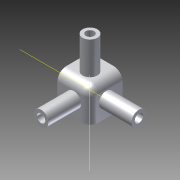
# Autodesk Inventor part: Corner
Saved by Autodesk Inventor 2011 (Build 150239000, 239)
## iProperties
Created: 2011-07-18
Part Number: Corner
Document SubType Name: Modeling
Designer: Seb Madgwick
Density: 1 g/cm^3
Author: Seb Madgwick
Autodesk Inventor part; units mm, degrees
ref_plane "YZ Plane" through (0, 0, 0) normal (1, 0, 0) x (0, 1, 0)
ref_plane "XZ Plane" through (0, 0, 0) normal (0, 1, 0) x (-1, 0, 0)
ref_plane "XY Plane" through (0, 0, 0) normal (0, 0, 1) x (1, 0, 0)
sketch "Sketch1" plane through (0, 0, 0) normal (0, 0, 1) x (1, 0, 0)
  line L0 (10, 10) -> (10, -10)
  line L1 (10, 10) -> (-10, 10)
  line L2 (-10, 10) -> (-10, -10)
  line L3 (-10, -10) -> (10, -10)
  point P0 (0, 0)
  dimension "d2" = 20
  dimension "d3" = 20
  dimension "d4" = 10
  dimension "d5" = 10
  constraints: 8 end point, 2 perpendicular, 1 parallel
  measures "d2" distance of L0.start L0.end
  measures "d3" distance of L0.start L1.end
  measures "d4" distance from line of L1 point (0, 0)
  measures "d5" distance from line of L2 point (0, 0)
extrude "Extrusion_main" add sketch "Sketch1" along normal mid plane 20
sketch "Sketch8" plane through (0, 0, 10) normal (0, 0, 1) x (1, 0, 0)
  circle A0 centre (0, 0) radius 2.55
  dimension "d31" = 5.1
  constraints: 1 centre point, 1 coincident
  measures "d31" diameter of A0
extrude "Extrusion_hole" cut sketch "Sketch8" against normal blind 7.5
sketch "Sketch9" plane through (0, 0, 10) normal (0, 0, 1) x (1, 0, 0)
  circle A0 centre (0, 0) radius 2.55 projected
  circle A1 centre (0, 0) radius 2.55
  circle A2 centre (0, 0) radius 4.55
  dimension "d34" = 5.1
  dimension "d35" = 9.1
  constraints: 2 centre point, 2 coincident, 1 concentric
  measures "d34" diameter of A1
  measures "d35" diameter of A2
extrude "Extrusion_sleeve" add sketch "Sketch9" along normal blind 20
ref_plane "Work Plane_frontTopNorm" through (-10, 10, 10) normal (0, 0.7071, -0.7071) x (1, 0, 0)
mirror "Mirror_top" about plane through (-10, 10, 10) normal (0, 0.7071, -0.7071) of "Extrusion_hole", "Extrusion_sleeve"
ref_plane "Work Plane_frontRightNorm" through (10, 10, 10) normal (0.7071, 0, -0.7071) x (0, -1, 0)
mirror "Mirror_right" about plane through (10, 10, 10) normal (0.7071, 0, -0.7071) of "Extrusion_hole", "Extrusion_sleeve"
fillet "Fillet_main" radius 5.45 3 edges at (10, 10, 0) (10, 0, 10) (0, 10, 10)
body "Solid1"
